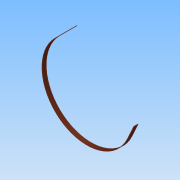
# Autodesk Inventor part: CopperContact
Saved by Autodesk Inventor 2017.3 (Build 213256000, 256)
## iProperties
Created: 2019-06-28
Part Number: CopperContact
Material: Copper, Alloy
Document SubType Name: Modeling
Designer: Derek Wider
Density: 8.92 g/cm^3
Appearance: Copper - Satin
Author: Derek Wider
Autodesk Inventor part; units mm, degrees
ref_plane "YZ Plane" through (0, 0, 0) normal (1, 0, 0) x (0, 1, 0)
ref_plane "XZ Plane" through (0, 0, 0) normal (0, 1, 0) x (-1, 0, 0)
ref_plane "XY Plane" through (0, 0, 0) normal (0, 0, 1) x (1, 0, 0)
sketch "Sketch1" plane through (0, 0, 0) normal (0, 0, 1) x (1, 0, 0)
  arc A0 (-16.164461, 16.164461) -> (20.718196, -9.661053) centre (0, 0) ccw
  arc A1 (-16.254264, 16.254264) -> (20.833297, -9.714726) centre (0, 0) ccw
  line L0 (-16.254264, 16.254264) -> (-16.164461, 16.164461)
  line L1 (20.718196, -9.661053) -> (20.833297, -9.714726)
  line L2 (0, 0) -> (15.160579, 0) construction
  line L3 (20.718196, -9.661053) -> (23.862711, -2.72013)
  line L4 (23.862711, -2.72013) -> (23.978386, -2.772535)
  line L5 (23.978386, -2.772535) -> (20.833297, -9.714726)
  line L6 (-16.254264, 16.254264) -> (-7.274007, 25.23452)
  line L7 (-7.274007, 25.23452) -> (-7.184205, 25.144717)
  line L8 (-7.184205, 25.144717) -> (-16.164461, 16.164461)
  line L9 (0, 0) -> (0, 16.116809) construction
  dimension "d0" = 45.72
  dimension "d1" = 45.974
  dimension "d2" = 25
  dimension "d3" = 7.62
  dimension "d5" = 12.7
  dimension "d6" = 45
  constraints: 20 end point, 4 point on circle, 3 perpendicular, 2 centre point, 2 coincident, 2 line through centre, 2 tangent, 1 horizontal, 1 vertical
  measures "d0" diameter of A0
  measures "d1" diameter of A1
  measures "d3" distance of L1.start L3.end
  measures "d5" distance of L0.start L6.end
sketch "Sketch1 outline for Extrusion1" plane through (0, 0, 0) normal (0, 0, 1) x (1, 0, 0)
  line L0 (-7.274007, 25.23452) -> (-16.254264, 16.254264)
  arc A0 (-16.254264, 16.254264) -> (20.833297, -9.714726) centre (0, 0) ccw
  line L1 (23.978386, -2.772535) -> (20.833297, -9.714726)
  line L2 (23.862711, -2.72013) -> (23.978386, -2.772535)
  line L3 (20.718196, -9.661053) -> (23.862711, -2.72013)
  arc A1 (20.718196, -9.661053) -> (-16.164461, 16.164461) centre (0, 0) cw
  line L4 (-16.164461, 16.164461) -> (-7.184205, 25.144717)
  line L5 (-7.184205, 25.144717) -> (-7.274007, 25.23452)
extrude "Extrusion1" add sketch "Sketch1 outline for Extrusion1" along normal blind 2.159
body "Solid1"
